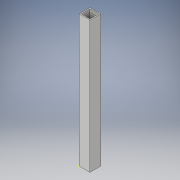
# Autodesk Inventor part: Control Panel Mount
Saved by Autodesk Inventor 2017 (Build 210142000, 142)
## iProperties
Created: 2020-02-07
Part Number: Control Panel Mount
Material: Generic
Document SubType Name: Modeling
Designer: S332862739
Density: 1 g/cm^3
Appearance: Default
Author: S332862739
Autodesk Inventor part; units mm, degrees
ref_plane "YZ Plane" through (0, 0, 0) normal (1, 0, 0) x (0, 1, 0)
ref_plane "XZ Plane" through (0, 0, 0) normal (0, 1, 0) x (-1, 0, 0)
ref_plane "XY Plane" through (0, 0, 0) normal (0, 0, 1) x (1, 0, 0)
sketch "Sketch1" plane through (0, 0, 0) normal (0, 1, 0) x (-1, 0, 0)
  line L0 (0, 0) -> (-25.4, 0)
  line L1 (-25.4, 0) -> (-25.4, -25.4)
  line L2 (-25.4, -25.4) -> (0, -25.4)
  line L3 (0, -25.4) -> (0, 0)
  dimension "d0" = 25.4
  dimension "d1" = 25.4
  constraints: 8 end point, 2 parallel, 1 horizontal, 1 perpendicular
  measures "d0" distance of L2.end L1.end
  measures "d1" distance of L1.end L0.end
extrude "Extrusion1" add sketch "Sketch1" along normal blind 307.975
sketch "Sketch4" plane through (0, 0, 0) normal (0, -1, 0) x (1, 0, 0)
  line L0 (22.86, -2.54) -> (2.54, -2.54)
  line L1 (2.54, -2.54) -> (2.54, -22.86)
  line L2 (2.54, -22.86) -> (22.86, -22.86)
  line L3 (22.86, -22.86) -> (22.86, -2.54)
  line L4 (25.4, 0) -> (25.4, -25.4) projected
  line L5 (25.4, -25.4) -> (0, -25.4) projected
  point P0 (0, 0)
  dimension "d13" = 20.32
  dimension "d14" = 20.32
  dimension "d15" = 2.54
  dimension "d16" = 2.54
  constraints: 8 end point, 2 parallel, 1 horizontal, 1 perpendicular
  measures "d13" distance of L2.end L1.end
  measures "d14" distance of L1.end L0.end
  measures "d15" distance between parallel lines of L3 L4
  measures "d16" distance between parallel lines of L2 L5
extrude "Extrusion4" cut sketch "Sketch4" against normal blind 448.31
sketch "Sketch15" plane through (0, 0, -25.4) normal (-1, 0, 0) x (0, 0, 1)
  point P0 (25.4, 0)
body "Solid1"
